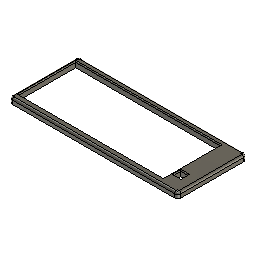
top (Autodesk Fusion 360 design; units mm, degrees)
part number: 2026-03-14-23-38-17-885
Autodesk Fusion 360 part; units mm, degrees
(part 1 of 2)
sketch "Sketch1" plane through (0, 0, 0) normal (0, 0, 1) x (1, 0, 0)
  line L0 (27.4732, 9.3182) -> (40.4732, 9.3182)
  line L1 (-101.1143, 52.4682) -> (-88.1143, 52.4682)
  line L2 (-96.3518, -9.7318) -> (-83.3518, -9.7318)
  arc A0 (-75.7081, -29.2818) -> (-76.2081, -28.7818) centre (-76.2081, -29.2818) ccw
  line L3 (127.4857, 66.4682) -> (140.4857, 66.4682)
  line L4 (146.5357, -4.6818) -> (159.5357, -4.6818)
  line L5 (160.0357, 8.8182) -> (160.0357, -4.1818)
  arc A1 (-40.4893, 14.3682) -> (-39.9893, 14.8682) centre (-40.4893, 14.8682) ccw
  line L6 (75.0982, -23.7318) -> (88.0982, -23.7318)
  arc A2 (146.5357, -28.7818) -> (146.0357, -29.2818) centre (146.5357, -29.2818) ccw
  arc A3 (140.9857, 65.9682) -> (140.4857, 66.4682) centre (140.4857, 65.9682) ccw
  line L7 (146.5357, -9.7318) -> (159.5357, -9.7318)
  arc A4 (36.2107, 27.8682) -> (35.7107, 28.3682) centre (35.7107, 27.8682) ccw
  arc A5 (-45.2518, -23.7318) -> (-44.7518, -23.2318) centre (-45.2518, -23.2318) ccw
  arc A6 (50.4982, -10.2318) -> (49.9982, -9.7318) centre (49.9982, -10.2318) ccw
  arc A7 (17.9482, -9.7318) -> (17.4482, -10.2318) centre (17.9482, -10.2318) ccw
  line L8 (3.6607, 28.3682) -> (16.6607, 28.3682)
  line L9 (8.4232, -4.6818) -> (21.4232, -4.6818)
  line L10 (13.1857, 47.4182) -> (26.1857, 47.4182)
  line L11 (13.1857, 33.4182) -> (26.1857, 33.4182)
  line L12 (3.6607, 14.3682) -> (16.6607, 14.3682)
  line L13 (212.5639, -64.1628) -> (-153.6501, -64.1628)
  line L14 (-153.6501, 86.0492) -> (212.5639, 86.0492)
  line L15 (187.5639, -17.1628) -> (187.5639, -32.1628)
  arc A8 (-44.7518, -10.2318) -> (-45.2518, -9.7318) centre (-45.2518, -10.2318) ccw
  arc A9 (-39.7018, -23.2318) -> (-39.2018, -23.7318) centre (-39.2018, -23.2318) ccw
  line L16 (70.3357, -42.7818) -> (83.3357, -42.7818)
  arc A10 (115.5794, 9.3182) -> (115.0794, 8.8182) centre (115.5794, 8.8182) ccw
  arc A11 (146.5357, 47.4182) -> (146.0357, 46.9182) centre (146.5357, 46.9182) ccw
  line L17 (172.5639, -32.1628) -> (172.5639, -17.1628)
  line L18 (26.6857, 46.9182) -> (26.6857, 33.9182)
  arc A12 (-49.2268, -4.1818) -> (-48.7268, -4.6818) centre (-48.7268, -4.1818) ccw
  circle A13 centre (207.0639, 80.5492) radius 1.45
  line L19 (-30.4643, 46.9182) -> (-30.4643, 33.9182)
  line L20 (3.6607, 52.4682) -> (16.6607, 52.4682)
  line L21 (3.6607, 66.4682) -> (16.6607, 66.4682)
  line L22 (-96.3518, -23.7318) -> (-83.3518, -23.7318)
  line L23 (-111.8701, -25.7318) -> (-105.8701, -25.7318)
  line L24 (-113.8081, -10.2318) -> (-113.8081, -23.2318)
  arc A14 (12.6857, 33.9182) -> (13.1857, 33.4182) centre (13.1857, 33.9182) ccw
  arc A15 (-89.2081, -28.7818) -> (-89.7081, -29.2818) centre (-89.2081, -29.2818) ccw
  arc A16 (-35.7268, -4.6818) -> (-35.2268, -4.1818) centre (-35.7268, -4.1818) ccw
  arc A17 (-15.3893, 28.3682) -> (-15.8893, 27.8682) centre (-15.3893, 27.8682) ccw
  line L25 (-6.3643, 46.9182) -> (-6.3643, 33.9182)
  line L26 (-136.2461, -11.2318) -> (-136.2461, -25.2318)
  line L27 (60.8107, 28.3682) -> (73.8107, 28.3682)
  arc A18 (-88.1143, 33.4182) -> (-87.6143, 33.9182) centre (-88.1143, 33.9182) ccw
  line L28 (69.8357, 46.9182) -> (69.8357, 33.9182)
  arc A19 (-39.2018, -9.7318) -> (-39.7018, -10.2318) centre (-39.2018, -10.2318) ccw
  line L29 (-44.4643, 46.9182) -> (-44.4643, 33.9182)
  arc A20 (-96.8518, -23.2318) -> (-96.3518, -23.7318) centre (-96.3518, -23.2318) ccw
  line L30 (-82.5643, 65.9682) -> (-82.5643, 52.9682)
  line L31 (101.2919, -23.7318) -> (114.2919, -23.7318)
  arc A21 (93.3607, 27.8682) -> (92.8607, 28.3682) centre (92.8607, 27.8682) ccw
  arc A22 (-123.3331, -29.2818) -> (-123.8331, -28.7818) centre (-123.8331, -29.2818) ccw
  line L32 (55.2607, 65.9682) -> (55.2607, 52.9682)
  arc A23 (-30.9643, 33.4182) -> (-30.4643, 33.9182) centre (-30.9643, 33.9182) ccw
  arc A24 (51.2857, 47.4182) -> (50.7857, 46.9182) centre (51.2857, 46.9182) ccw
  line L33 (-30.1768, 8.8182) -> (-30.1768, -4.1818)
  line L34 (88.8857, 65.9682) -> (88.8857, 52.9682)
  line L35 (-129.2461, -11.2318) -> (-129.2461, -25.2318)
  line L36 (-112.3701, -11.2318) -> (-112.3701, -25.2318)
  circle A25 centre (-148.1501, -58.6628) radius 1.45
  arc A26 (17.1607, 27.8682) -> (16.6607, 28.3682) centre (16.6607, 27.8682) ccw
  arc A27 (-106.3768, -4.1818) -> (-105.8768, -4.6818) centre (-105.8768, -4.1818) ccw
  arc A28 (-54.7768, -4.6818) -> (-54.2768, -4.1818) centre (-54.7768, -4.1818) ccw
  arc A29 (-50.0143, 33.4182) -> (-49.5143, 33.9182) centre (-50.0143, 33.9182) ccw
  line L37 (-86.8268, 9.3182) -> (-73.8268, 9.3182)
  arc A30 (127.4857, 66.4682) -> (126.9857, 65.9682) centre (127.4857, 65.9682) ccw
  arc A31 (7.6357, 46.9182) -> (7.1357, 47.4182) centre (7.1357, 46.9182) ccw
  line L38 (-106.6643, 46.9182) -> (-106.6643, 33.9182)
  arc A32 (89.3857, 47.4182) -> (88.8857, 46.9182) centre (89.3857, 46.9182) ccw
  arc A33 (160.0357, -29.2818) -> (159.5357, -28.7818) centre (159.5357, -29.2818) ccw
  arc A34 (106.6414, -6.1818) -> (107.1414, -6.6818) centre (107.1414, -6.1818) ccw
  line L39 (127.4857, 52.4682) -> (140.4857, 52.4682)
  arc A35 (-77.3018, -9.7318) -> (-77.8018, -10.2318) centre (-77.3018, -10.2318) ccw
  line L40 (40.9732, 8.8182) -> (40.9732, -4.1818)
  line L41 (8.4232, 9.3182) -> (21.4232, 9.3182)
  arc A36 (26.9732, -4.1818) -> (27.4732, -4.6818) centre (27.4732, -4.1818) ccw
  arc A37 (40.9732, 8.8182) -> (40.4732, 9.3182) centre (40.4732, 8.8182) ccw
  arc A38 (-111.8701, -10.7318) -> (-112.3701, -11.2318) centre (-111.8701, -11.2318) ccw
  line L42 (-134.9518, 27.8682) -> (-134.9518, 14.8682)
  arc A39 (-35.2268, 8.8182) -> (-35.7268, 9.3182) centre (-35.7268, 8.8182) ccw
  arc A40 (-120.6643, 33.9182) -> (-120.1643, 33.4182) centre (-120.1643, 33.9182) ccw
  arc A41 (-64.3018, -23.7318) -> (-63.8018, -23.2318) centre (-64.3018, -23.2318) ccw
  arc A42 (-43.9643, 47.4182) -> (-44.4643, 46.9182) centre (-43.9643, 46.9182) ccw
  arc A43 (-101.1143, 66.4682) -> (-101.6143, 65.9682) centre (-101.1143, 65.9682) ccw
  arc A44 (-134.9518, 14.8682) -> (-134.4518, 14.3682) centre (-134.4518, 14.8682) ccw
  arc A45 (-113.8081, -10.2318) -> (-114.3081, -9.7318) centre (-114.3081, -10.2318) ccw
  line L43 (17.1607, 65.9682) -> (17.1607, 52.9682)
  arc A46 (7.1357, 33.4182) -> (7.6357, 33.9182) centre (7.1357, 33.9182) ccw
  arc A47 (-53.4893, 28.3682) -> (-53.9893, 27.8682) centre (-53.4893, 27.8682) ccw
  line L44 (-111.8701, -10.7318) -> (-105.8701, -10.7318)
  arc A48 (98.1232, 8.8182) -> (97.6232, 9.3182) centre (97.6232, 8.8182) ccw
  arc A49 (-125.7143, 65.9682) -> (-126.2143, 66.4682) centre (-126.2143, 65.9682) ccw
  arc A50 (108.4357, -28.7818) -> (107.9357, -29.2818) centre (108.4357, -29.2818) ccw
  line L45 (-15.3893, 66.4682) -> (-2.3893, 66.4682)
  line L46 (-101.6143, 65.9682) -> (-101.6143, 52.9682)
  arc A51 (79.8607, 28.3682) -> (79.3607, 27.8682) centre (79.8607, 27.8682) ccw
  line L47 (-44.4643, 65.9682) -> (-44.4643, 52.9682)
  arc A52 (-63.5143, 33.9182) -> (-63.0143, 33.4182) centre (-63.0143, 33.9182) ccw
  line L48 (-78.0893, 27.8682) -> (-78.0893, 14.8682)
  arc A53 (17.1607, 65.9682) -> (16.6607, 66.4682) centre (16.6607, 65.9682) ccw
  line L49 (-53.4893, 28.3682) -> (-40.4893, 28.3682)
  line L50 (-89.2081, -42.7818) -> (-76.2081, -42.7818)
  arc A54 (-64.2706, -29.7818) -> (-64.7706, -30.2818) centre (-64.2706, -30.2818) ccw
  arc A55 (88.8857, 52.9682) -> (89.3857, 52.4682) centre (89.3857, 52.9682) ccw
  arc A56 (-50.0143, 52.4682) -> (-49.5143, 52.9682) centre (-50.0143, 52.9682) ccw
  line L51 (-43.9643, 66.4682) -> (-30.9643, 66.4682)
  line L52 (-82.0643, 52.4682) -> (-69.0643, 52.4682)
  line L53 (-139.2143, 66.4682) -> (-126.2143, 66.4682)
  arc A57 (-15.8893, 52.9682) -> (-15.3893, 52.4682) centre (-15.3893, 52.9682) ccw
  arc A58 (55.2607, 65.9682) -> (54.7607, 66.4682) centre (54.7607, 65.9682) ccw
  line L54 (-73.0393, 27.8682) -> (-73.0393, 14.8682)
  arc A59 (-24.9143, 47.4182) -> (-25.4143, 46.9182) centre (-24.9143, 46.9182) ccw
  arc A60 (83.3357, 33.4182) -> (83.8357, 33.9182) centre (83.3357, 33.9182) ccw
  arc A61 (-120.1643, 47.4182) -> (-120.6643, 46.9182) centre (-120.1643, 46.9182) ccw
  line L55 (-139.2143, 47.4182) -> (-126.2143, 47.4182)
  arc A62 (-72.5393, 28.3682) -> (-73.0393, 27.8682) centre (-72.5393, 27.8682) ccw
  line L56 (-63.5143, 65.9682) -> (-63.5143, 52.9682)
  arc A63 (-82.5643, 33.9182) -> (-82.0643, 33.4182) centre (-82.0643, 33.9182) ccw
  line L57 (-139.7143, 65.9682) -> (-139.7143, 52.9682)
  arc A64 (-97.6393, 14.3682) -> (-97.1393, 14.8682) centre (-97.6393, 14.8682) ccw
  circle A65 centre (-148.1501, 80.5492) radius 1.45
  arc A66 (-68.5643, 46.9182) -> (-69.0643, 47.4182) centre (-69.0643, 46.9182) ccw
  line L58 (-82.0643, 47.4182) -> (-69.0643, 47.4182)
  arc A67 (-111.1393, 14.8682) -> (-110.6393, 14.3682) centre (-110.6393, 14.8682) ccw
  line L59 (7.6357, 46.9182) -> (7.6357, 33.9182)
  arc A68 (-49.5143, 65.9682) -> (-50.0143, 66.4682) centre (-50.0143, 65.9682) ccw
  arc A69 (-106.6643, 46.9182) -> (-107.1643, 47.4182) centre (-107.1643, 46.9182) ccw
  arc A70 (-20.9393, 27.8682) -> (-21.4393, 28.3682) centre (-21.4393, 27.8682) ccw
  arc A71 (-6.3643, 33.9182) -> (-5.8643, 33.4182) centre (-5.8643, 33.9182) ccw
  arc A72 (69.8357, 33.9182) -> (70.3357, 33.4182) centre (70.3357, 33.9182) ccw
  arc A73 (-107.1643, 33.4182) -> (-106.6643, 33.9182) centre (-107.1643, 33.9182) ccw
  arc A74 (7.9232, -4.1818) -> (8.4232, -4.6818) centre (8.4232, -4.1818) ccw
  arc A75 (55.5482, -23.2318) -> (56.0482, -23.7318) centre (56.0482, -23.2318) ccw
  arc A76 (51.2857, -28.7818) -> (50.7857, -29.2818) centre (51.2857, -29.2818) ccw
  arc A77 (-16.1768, 8.8182) -> (-16.6768, 9.3182) centre (-16.6768, 8.8182) ccw
  line L60 (35.7294, -44.7818) -> (41.7294, -44.7818)
  arc A78 (-21.4393, 14.3682) -> (-20.9393, 14.8682) centre (-21.4393, 14.8682) ccw
  line L61 (17.9482, -23.7318) -> (30.9482, -23.7318)
  line L62 (-16.1768, 8.8182) -> (-16.1768, -4.1818)
  line L63 (42.2294, -30.2818) -> (42.2294, -44.2818)
  arc A79 (-10.6268, 9.3182) -> (-11.1268, 8.8182) centre (-10.6268, 8.8182) ccw
  line L64 (84.6232, -4.6818) -> (97.6232, -4.6818)
  arc A80 (49.9982, -23.7318) -> (50.4982, -23.2318) centre (49.9982, -23.2318) ccw
  arc A81 (36.4982, -23.2318) -> (36.9982, -23.7318) centre (36.9982, -23.2318) ccw
  arc A82 (-6.6518, -10.2318) -> (-7.1518, -9.7318) centre (-7.1518, -10.2318) ccw
  line L65 (89.3857, 33.4182) -> (102.3857, 33.4182)
  line L66 (-67.7768, -4.6818) -> (-54.7768, -4.6818)
  line L67 (26.9732, 8.8182) -> (26.9732, -4.1818)
  arc A83 (31.4482, -10.2318) -> (30.9482, -9.7318) centre (30.9482, -10.2318) ccw
  arc A84 (46.5232, 9.3182) -> (46.0232, 8.8182) centre (46.5232, 8.8182) ccw
  arc A85 (22.2107, 14.8682) -> (22.7107, 14.3682) centre (22.7107, 14.8682) ccw
  line L68 (21.9232, 8.8182) -> (21.9232, -4.1818)
  line L69 (-135.7461, -25.7318) -> (-129.7461, -25.7318)
  arc A86 (64.2857, 33.4182) -> (64.7857, 33.9182) centre (64.2857, 33.9182) ccw
  arc A87 (-83.3518, -23.7318) -> (-82.8518, -23.2318) centre (-83.3518, -23.2318) ccw
  line L70 (-123.3331, -29.2818) -> (-123.3331, -42.2818)
  line L71 (-136.8331, -28.7818) -> (-123.8331, -28.7818)
  arc A88 (-89.7081, -42.2818) -> (-89.2081, -42.7818) centre (-89.2081, -42.2818) ccw
  line L72 (-127.8081, -10.2318) -> (-127.8081, -23.2318)
  arc A89 (89.3857, 66.4682) -> (88.8857, 65.9682) centre (89.3857, 65.9682) ccw
  arc A90 (101.2919, -9.7318) -> (100.7919, -10.2318) centre (101.2919, -10.2318) ccw
  arc A91 (41.7607, 66.4682) -> (41.2607, 65.9682) centre (41.7607, 65.9682) ccw
  line L73 (-82.0643, 66.4682) -> (-69.0643, 66.4682)
  arc A92 (-30.4643, 65.9682) -> (-30.9643, 66.4682) centre (-30.9643, 65.9682) ccw
  line L74 (-139.2143, 52.4682) -> (-126.2143, 52.4682)
  line L75 (-120.1643, 47.4182) -> (-107.1643, 47.4182)
  line L76 (22.2107, 65.9682) -> (22.2107, 52.9682)
  arc A93 (-29.6768, 9.3182) -> (-30.1768, 8.8182) centre (-29.6768, 8.8182) ccw
  line L77 (-110.6393, 28.3682) -> (-97.6393, 28.3682)
  arc A94 (-105.8768, 9.3182) -> (-106.3768, 8.8182) centre (-105.8768, 8.8182) ccw
  arc A95 (54.7607, 52.4682) -> (55.2607, 52.9682) centre (54.7607, 52.9682) ccw
  line L78 (-48.7268, 9.3182) -> (-35.7268, 9.3182)
  line L79 (-92.0893, 27.8682) -> (-92.0893, 14.8682)
  line L80 (-1.8893, 65.9682) -> (-1.8893, 52.9682)
  arc A96 (-76.2081, -42.7818) -> (-75.7081, -42.2818) centre (-76.2081, -42.2818) ccw
  arc A97 (-49.5143, 46.9182) -> (-50.0143, 47.4182) centre (-50.0143, 46.9182) ccw
  arc A98 (-129.2461, -11.2318) -> (-129.7461, -10.7318) centre (-129.7461, -11.2318) ccw
  arc A99 (-44.4643, 33.9182) -> (-43.9643, 33.4182) centre (-43.9643, 33.9182) ccw
  line L81 (83.8357, 65.9682) -> (83.8357, 52.9682)
  arc A100 (89.3857, -28.7818) -> (88.8857, -29.2818) centre (89.3857, -29.2818) ccw
  line L82 (-77.3018, -9.7318) -> (-64.3018, -9.7318)
  arc A101 (-135.7461, -10.7318) -> (-136.2461, -11.2318) centre (-135.7461, -11.2318) ccw
  circle A102 centre (207.0639, -58.6628) radius 1.45
  line L83 (22.7107, 28.3682) -> (35.7107, 28.3682)
  line L84 (-11.4143, 46.9182) -> (-11.4143, 33.9182)
  arc A103 (-1.8893, 65.9682) -> (-2.3893, 66.4682) centre (-2.3893, 65.9682) ccw
  arc A104 (70.3357, 47.4182) -> (69.8357, 46.9182) centre (70.3357, 46.9182) ccw
  arc A105 (64.2857, -42.7818) -> (64.7857, -42.2818) centre (64.2857, -42.2818) ccw
  line L85 (-105.3701, -11.2318) -> (-105.3701, -25.2318)
  line L86 (131.0174, -6.6818) -> (137.0174, -6.6818)
  line L87 (-58.2518, -9.7318) -> (-45.2518, -9.7318)
  line L88 (-101.1143, 33.4182) -> (-88.1143, 33.4182)
  line L89 (-120.9518, 27.8682) -> (-120.9518, 14.8682)
  arc A106 (-101.1143, 47.4182) -> (-101.6143, 46.9182) centre (-101.1143, 46.9182) ccw
  line L90 (-139.2143, 33.4182) -> (-126.2143, 33.4182)
  arc A107 (-110.6393, 28.3682) -> (-111.1393, 27.8682) centre (-110.6393, 27.8682) ccw
  line L91 (12.6857, 46.9182) -> (12.6857, 33.9182)
  arc A108 (-82.0643, 66.4682) -> (-82.5643, 65.9682) centre (-82.0643, 65.9682) ccw
  line L92 (-132.0706, 9.3182) -> (-119.0706, 9.3182)
  arc A109 (-120.9518, 27.8682) -> (-121.4518, 28.3682) centre (-121.4518, 27.8682) ccw
  arc A110 (-125.7143, 46.9182) -> (-126.2143, 47.4182) centre (-126.2143, 46.9182) ccw
  arc A111 (-139.7143, 33.9182) -> (-139.2143, 33.4182) centre (-139.2143, 33.9182) ccw
  arc A112 (-97.1393, 27.8682) -> (-97.6393, 28.3682) centre (-97.6393, 27.8682) ccw
  arc A113 (-2.3893, 14.3682) -> (-1.8893, 14.8682) centre (-2.3893, 14.8682) ccw
  arc A114 (35.2294, -44.2818) -> (35.7294, -44.7818) centre (35.7294, -44.2818) ccw
  arc A115 (-11.1268, -4.1818) -> (-10.6268, -4.6818) centre (-10.6268, -4.1818) ccw
  arc A116 (50.7857, -42.2818) -> (51.2857, -42.7818) centre (51.2857, -42.2818) ccw
  line L93 (41.7607, 14.3682) -> (54.7607, 14.3682)
  arc A117 (35.7294, -29.7818) -> (35.2294, -30.2818) centre (35.7294, -30.2818) ccw
  arc A118 (-20.1518, -9.7318) -> (-20.6518, -10.2318) centre (-20.1518, -10.2318) ccw
  arc A119 (8.4232, 9.3182) -> (7.9232, 8.8182) centre (8.4232, 8.8182) ccw
  line L94 (35.2294, -30.2818) -> (35.2294, -44.2818)
  line L95 (89.3857, 66.4682) -> (102.3857, 66.4682)
  line L96 (-1.1018, -9.7318) -> (11.8982, -9.7318)
  line L97 (36.9982, -23.7318) -> (49.9982, -23.7318)
  line L98 (36.4982, -10.2318) -> (36.4982, -23.2318)
  line L99 (55.5482, -10.2318) -> (55.5482, -23.2318)
  line L100 (-11.1268, 8.8182) -> (-11.1268, -4.1818)
  line L101 (7.9232, 8.8182) -> (7.9232, -4.1818)
  arc A120 (17.4482, -23.2318) -> (17.9482, -23.7318) centre (17.9482, -23.2318) ccw
  arc A121 (3.1607, 14.8682) -> (3.6607, 14.3682) centre (3.6607, 14.8682) ccw
  line L102 (-15.3893, 14.3682) -> (-2.3893, 14.3682)
  arc A122 (-15.8893, 14.8682) -> (-15.3893, 14.3682) centre (-15.3893, 14.8682) ccw
  line L103 (50.7857, -29.2818) -> (50.7857, -42.2818)
  arc A123 (30.9482, -23.7318) -> (31.4482, -23.2318) centre (30.9482, -23.2318) ccw
  line L104 (27.4732, -4.6818) -> (40.4732, -4.6818)
  line L105 (88.8857, -29.2818) -> (88.8857, -42.2818)
  arc A124 (69.8357, -42.2818) -> (70.3357, -42.7818) centre (70.3357, -42.2818) ccw
  line L106 (-125.7143, 46.9182) -> (-125.7143, 33.9182)
  line L107 (-48.7268, -4.6818) -> (-35.7268, -4.6818)
  arc A125 (3.6607, 66.4682) -> (3.1607, 65.9682) centre (3.6607, 65.9682) ccw
  arc A126 (-68.2768, -4.1818) -> (-67.7768, -4.6818) centre (-67.7768, -4.1818) ccw
  line L108 (146.5357, -42.7818) -> (159.5357, -42.7818)
  arc A127 (-105.3701, -11.2318) -> (-105.8701, -10.7318) centre (-105.8701, -11.2318) ccw
  arc A128 (13.1857, 47.4182) -> (12.6857, 46.9182) centre (13.1857, 46.9182) ccw
  arc A129 (32.2357, 47.4182) -> (31.7357, 46.9182) centre (32.2357, 46.9182) ccw
  arc A130 (113.1414, -6.6818) -> (113.6414, -6.1818) centre (113.1414, -6.1818) ccw
  arc A131 (26.6857, 46.9182) -> (26.1857, 47.4182) centre (26.1857, 46.9182) ccw
  arc A132 (-34.4393, 28.3682) -> (-34.9393, 27.8682) centre (-34.4393, 27.8682) ccw
  line L109 (-68.5643, 46.9182) -> (-68.5643, 33.9182)
  line L110 (127.4857, -23.7318) -> (140.4857, -23.7318)
  arc A133 (83.8357, 46.9182) -> (83.3357, 47.4182) centre (83.3357, 46.9182) ccw
  arc A134 (64.7857, 46.9182) -> (64.2857, 47.4182) centre (64.2857, 46.9182) ccw
  line L111 (108.4357, -42.7818) -> (121.4357, -42.7818)
  arc A135 (140.4857, -42.7818) -> (140.9857, -42.2818) centre (140.4857, -42.2818) ccw
  line L112 (64.7857, -29.2818) -> (64.7857, -42.2818)
  line L113 (146.5357, -28.7818) -> (159.5357, -28.7818)
  arc A136 (-77.8018, -23.2318) -> (-77.3018, -23.7318) centre (-77.3018, -23.2318) ccw
  arc A137 (-99.5206, -29.2818) -> (-100.0206, -28.7818) centre (-100.0206, -29.2818) ccw
  line L114 (-91.5893, 14.3682) -> (-78.5893, 14.3682)
  arc A138 (31.7357, 33.9182) -> (32.2357, 33.4182) centre (32.2357, 33.9182) ccw
  line L115 (-127.3081, -23.7318) -> (-114.3081, -23.7318)
  line L116 (-15.3893, 28.3682) -> (-2.3893, 28.3682)
  arc A139 (-25.4143, 33.9182) -> (-24.9143, 33.4182) centre (-24.9143, 33.9182) ccw
  line L117 (-111.1393, 27.8682) -> (-111.1393, 14.8682)
  arc A140 (-118.5706, 8.8182) -> (-119.0706, 9.3182) centre (-119.0706, 8.8182) ccw
  arc A141 (55.2607, 27.8682) -> (54.7607, 28.3682) centre (54.7607, 27.8682) ccw
  arc A142 (-87.6143, 65.9682) -> (-88.1143, 66.4682) centre (-88.1143, 65.9682) ccw
  line L118 (-120.1643, 33.4182) -> (-107.1643, 33.4182)
  arc A143 (-139.2143, 66.4682) -> (-139.7143, 65.9682) centre (-139.2143, 65.9682) ccw
  arc A144 (-139.7143, 52.9682) -> (-139.2143, 52.4682) centre (-139.2143, 52.9682) ccw
  line L119 (41.2607, 65.9682) -> (41.2607, 52.9682)
  line L120 (69.8357, 65.9682) -> (69.8357, 52.9682)
  arc A145 (-101.6143, 52.9682) -> (-101.1143, 52.4682) centre (-101.1143, 52.9682) ccw
  line L121 (70.3357, 47.4182) -> (83.3357, 47.4182)
  arc A146 (36.2107, 65.9682) -> (35.7107, 66.4682) centre (35.7107, 65.9682) ccw
  arc A147 (3.1607, 52.9682) -> (3.6607, 52.4682) centre (3.6607, 52.9682) ccw
  arc A148 (-82.5643, 52.9682) -> (-82.0643, 52.4682) centre (-82.0643, 52.9682) ccw
  line L122 (22.7107, 52.4682) -> (35.7107, 52.4682)
  line L123 (70.3357, 33.4182) -> (83.3357, 33.4182)
  arc A149 (-15.3893, 66.4682) -> (-15.8893, 65.9682) centre (-15.3893, 65.9682) ccw
  arc A150 (-91.5893, 28.3682) -> (-92.0893, 27.8682) centre (-91.5893, 27.8682) ccw
  arc A151 (-126.2143, 52.4682) -> (-125.7143, 52.9682) centre (-126.2143, 52.9682) ccw
  arc A152 (-132.0706, 9.3182) -> (-132.5706, 8.8182) centre (-132.0706, 8.8182) ccw
  arc A153 (3.6607, 28.3682) -> (3.1607, 27.8682) centre (3.6607, 27.8682) ccw
  arc A154 (-78.0893, 27.8682) -> (-78.5893, 28.3682) centre (-78.5893, 27.8682) ccw
  arc A155 (-30.4643, 46.9182) -> (-30.9643, 47.4182) centre (-30.9643, 46.9182) ccw
  arc A156 (69.8357, 52.9682) -> (70.3357, 52.4682) centre (70.3357, 52.9682) ccw
  arc A157 (-87.6143, 46.9182) -> (-88.1143, 47.4182) centre (-88.1143, 46.9182) ccw
  arc A158 (16.6607, 14.3682) -> (17.1607, 14.8682) centre (16.6607, 14.8682) ccw
  arc A159 (40.4732, -4.6818) -> (40.9732, -4.1818) centre (40.4732, -4.1818) ccw
  arc A160 (27.4732, 9.3182) -> (26.9732, 8.8182) centre (27.4732, 8.8182) ccw
  line L124 (22.7107, 14.3682) -> (35.7107, 14.3682)
  arc A161 (126.9857, -23.2318) -> (127.4857, -23.7318) centre (127.4857, -23.2318) ccw
  arc A162 (-57.7706, -30.2818) -> (-58.2706, -29.7818) centre (-58.2706, -30.2818) ccw
  line L125 (31.7357, 46.9182) -> (31.7357, 33.9182)
  arc A163 (127.4857, -9.7318) -> (126.9857, -10.2318) centre (127.4857, -10.2318) ccw
  line L126 (-58.2518, -23.7318) -> (-45.2518, -23.7318)
  arc A164 (-58.2706, -44.7818) -> (-57.7706, -44.2818) centre (-58.2706, -44.2818) ccw
  line L127 (146.5357, 47.4182) -> (159.5357, 47.4182)
  arc A165 (126.9857, 52.9682) -> (127.4857, 52.4682) centre (127.4857, 52.9682) ccw
  arc A166 (-73.0393, 14.8682) -> (-72.5393, 14.3682) centre (-72.5393, 14.8682) ccw
  arc A167 (70.3357, -28.7818) -> (69.8357, -29.2818) centre (70.3357, -29.2818) ccw
  line L128 (-86.8268, -4.6818) -> (-73.8268, -4.6818)
  line L129 (-54.2768, 8.8182) -> (-54.2768, -4.1818)
  arc A168 (-63.8018, -10.2318) -> (-64.3018, -9.7318) centre (-64.3018, -10.2318) ccw
  arc A169 (-101.6143, 33.9182) -> (-101.1143, 33.4182) centre (-101.1143, 33.9182) ccw
  arc A170 (-63.5143, 52.9682) -> (-63.0143, 52.4682) centre (-63.0143, 52.9682) ccw
  arc A171 (16.6607, 52.4682) -> (17.1607, 52.9682) centre (16.6607, 52.9682) ccw
  line L130 (-97.1393, 27.8682) -> (-97.1393, 14.8682)
  line L131 (-49.5143, 46.9182) -> (-49.5143, 33.9182)
  line L132 (-82.0643, 33.4182) -> (-69.0643, 33.4182)
  arc A172 (-82.0643, 47.4182) -> (-82.5643, 46.9182) centre (-82.0643, 46.9182) ccw
  arc A173 (-126.2143, 33.4182) -> (-125.7143, 33.9182) centre (-126.2143, 33.9182) ccw
  arc A174 (-64.7706, -44.2818) -> (-64.2706, -44.7818) centre (-64.2706, -44.2818) ccw
  arc A175 (-11.9143, 33.4182) -> (-11.4143, 33.9182) centre (-11.9143, 33.9182) ccw
  line L133 (-134.4518, 28.3682) -> (-121.4518, 28.3682)
  line L134 (-43.9643, 52.4682) -> (-30.9643, 52.4682)
  arc A176 (-92.3768, 8.8182) -> (-92.8768, 9.3182) centre (-92.8768, 8.8182) ccw
  line L135 (22.7107, 66.4682) -> (35.7107, 66.4682)
  line L136 (-5.8643, 33.4182) -> (7.1357, 33.4182)
  line L137 (70.3357, 66.4682) -> (83.3357, 66.4682)
  line L138 (-43.9643, 47.4182) -> (-30.9643, 47.4182)
  line L139 (-89.7081, -29.2818) -> (-89.7081, -42.2818)
  line L140 (64.7857, 46.9182) -> (64.7857, 33.9182)
  arc A177 (-139.2143, 47.4182) -> (-139.7143, 46.9182) centre (-139.2143, 46.9182) ccw
  arc A178 (-63.0143, 47.4182) -> (-63.5143, 46.9182) centre (-63.0143, 46.9182) ccw
  line L141 (3.1607, 65.9682) -> (3.1607, 52.9682)
  arc A179 (-78.5893, 14.3682) -> (-78.0893, 14.8682) centre (-78.5893, 14.8682) ccw
  line L142 (107.9357, -29.2818) -> (107.9357, -42.2818)
  line L143 (-135.7461, -10.7318) -> (-129.7461, -10.7318)
  arc A180 (60.8107, 28.3682) -> (60.3107, 27.8682) centre (60.8107, 27.8682) ccw
  arc A181 (35.7107, 52.4682) -> (36.2107, 52.9682) centre (35.7107, 52.9682) ccw
  line L144 (46.0232, 8.8182) -> (46.0232, -4.1818)
  arc A182 (35.7107, 14.3682) -> (36.2107, 14.8682) centre (35.7107, 14.8682) ccw
  line L145 (101.2919, -9.7318) -> (114.2919, -9.7318)
  arc A183 (102.3857, -42.7818) -> (102.8857, -42.2818) centre (102.3857, -42.2818) ccw
  line L146 (146.5357, -23.7318) -> (159.5357, -23.7318)
  arc A184 (-82.8518, -10.2318) -> (-83.3518, -9.7318) centre (-83.3518, -10.2318) ccw
  arc A185 (-119.0706, -4.6818) -> (-118.5706, -4.1818) centre (-119.0706, -4.1818) ccw
  arc A186 (-136.8331, -28.7818) -> (-137.3331, -29.2818) centre (-136.8331, -29.2818) ccw
  arc A187 (140.4857, 52.4682) -> (140.9857, 52.9682) centre (140.4857, 52.9682) ccw
  line L147 (70.3357, -28.7818) -> (83.3357, -28.7818)
  line L148 (-113.5206, -29.2818) -> (-113.5206, -42.2818)
  arc A188 (22.7107, 28.3682) -> (22.2107, 27.8682) centre (22.7107, 27.8682) ccw
  arc A189 (-54.2768, 8.8182) -> (-54.7768, 9.3182) centre (-54.7768, 8.8182) ccw
  arc A190 (64.7857, -29.2818) -> (64.2857, -28.7818) centre (64.2857, -29.2818) ccw
  line L149 (115.0794, 8.8182) -> (115.0794, -4.1818)
  arc A191 (-123.8331, -42.7818) -> (-123.3331, -42.2818) centre (-123.8331, -42.2818) ccw
  arc A192 (-1.8893, 27.8682) -> (-2.3893, 28.3682) centre (-2.3893, 27.8682) ccw
  arc A193 (-132.5706, -4.1818) -> (-132.0706, -4.6818) centre (-132.0706, -4.1818) ccw
  arc A194 (-2.3893, 52.4682) -> (-1.8893, 52.9682) centre (-2.3893, 52.9682) ccw
  arc A195 (-59.0393, 27.8682) -> (-59.5393, 28.3682) centre (-59.5393, 27.8682) ccw
  arc A196 (-113.0206, -28.7818) -> (-113.5206, -29.2818) centre (-113.0206, -29.2818) ccw
  arc A197 (45.7357, 46.9182) -> (45.2357, 47.4182) centre (45.2357, 46.9182) ccw
  arc A198 (-100.0206, -42.7818) -> (-99.5206, -42.2818) centre (-100.0206, -42.2818) ccw
  arc A199 (-127.3081, -9.7318) -> (-127.8081, -10.2318) centre (-127.3081, -10.2318) ccw
  line L150 (-49.2268, 8.8182) -> (-49.2268, -4.1818)
  arc A200 (140.4857, -23.7318) -> (140.9857, -23.2318) centre (140.4857, -23.2318) ccw
  arc A201 (-59.5393, 14.3682) -> (-59.0393, 14.8682) centre (-59.5393, 14.8682) ccw
  arc A202 (26.1857, 33.4182) -> (26.6857, 33.9182) centre (26.1857, 33.9182) ccw
  arc A203 (-11.4143, 46.9182) -> (-11.9143, 47.4182) centre (-11.9143, 46.9182) ccw
  line L151 (-63.5143, 46.9182) -> (-63.5143, 33.9182)
  arc A204 (-127.8081, -23.2318) -> (-127.3081, -23.7318) centre (-127.3081, -23.2318) ccw
  line L152 (102.8857, -29.2818) -> (102.8857, -42.2818)
  arc A205 (114.7919, -10.2318) -> (114.2919, -9.7318) centre (114.2919, -10.2318) ccw
  arc A206 (-58.2518, -9.7318) -> (-58.7518, -10.2318) centre (-58.2518, -10.2318) ccw
  arc A207 (-113.5206, -42.2818) -> (-113.0206, -42.7818) centre (-113.0206, -42.2818) ccw
  line L153 (-99.5206, -29.2818) -> (-99.5206, -42.2818)
  arc A208 (-67.7768, 9.3182) -> (-68.2768, 8.8182) centre (-67.7768, 8.8182) ccw
  line L154 (-87.6143, 46.9182) -> (-87.6143, 33.9182)
  line L155 (-82.5643, 46.9182) -> (-82.5643, 33.9182)
  line L156 (-120.6643, 46.9182) -> (-120.6643, 33.9182)
  arc A209 (159.5357, -23.7318) -> (160.0357, -23.2318) centre (159.5357, -23.2318) ccw
  line L157 (-137.3331, -29.2818) -> (-137.3331, -42.2818)
  arc A210 (74.3107, 27.8682) -> (73.8107, 28.3682) centre (73.8107, 27.8682) ccw
  line L158 (-49.5143, 65.9682) -> (-49.5143, 52.9682)
  line L159 (36.2107, 65.9682) -> (36.2107, 52.9682)
  line L160 (79.8607, 28.3682) -> (92.8607, 28.3682)
  arc A211 (22.7107, 66.4682) -> (22.2107, 65.9682) centre (22.7107, 65.9682) ccw
  line L161 (-125.7143, 65.9682) -> (-125.7143, 52.9682)
  arc A212 (-134.4518, 28.3682) -> (-134.9518, 27.8682) centre (-134.4518, 27.8682) ccw
  arc A213 (-5.8643, 47.4182) -> (-6.3643, 46.9182) centre (-5.8643, 46.9182) ccw
  arc A214 (-121.4518, 14.3682) -> (-120.9518, 14.8682) centre (-121.4518, 14.8682) ccw
  arc A215 (-88.1143, 52.4682) -> (-87.6143, 52.9682) centre (-88.1143, 52.9682) ccw
  line L162 (-68.5643, 65.9682) -> (-68.5643, 52.9682)
  line L163 (-110.6393, 14.3682) -> (-97.6393, 14.3682)
  line L164 (70.3357, 52.4682) -> (83.3357, 52.4682)
  line L165 (-134.4518, 14.3682) -> (-121.4518, 14.3682)
  arc A216 (88.8857, 33.9182) -> (89.3857, 33.4182) centre (89.3857, 33.9182) ccw
  arc A217 (41.2607, 52.9682) -> (41.7607, 52.4682) centre (41.7607, 52.9682) ccw
  line L166 (88.8857, 46.9182) -> (88.8857, 33.9182)
  line L167 (83.8357, 46.9182) -> (83.8357, 33.9182)
  line L168 (-5.8643, 47.4182) -> (7.1357, 47.4182)
  arc A218 (-43.9643, 66.4682) -> (-44.4643, 65.9682) centre (-43.9643, 65.9682) ccw
  arc A219 (22.2107, 52.9682) -> (22.7107, 52.4682) centre (22.7107, 52.9682) ccw
  line L169 (113.6414, 7.8182) -> (113.6414, -6.1818)
  arc A220 (-63.0143, 66.4682) -> (-63.5143, 65.9682) centre (-63.0143, 65.9682) ccw
  arc A221 (-69.0643, 52.4682) -> (-68.5643, 52.9682) centre (-69.0643, 52.9682) ccw
  line L170 (-87.6143, 65.9682) -> (-87.6143, 52.9682)
  line L171 (-91.5893, 28.3682) -> (-78.5893, 28.3682)
  arc A222 (70.3357, 66.4682) -> (69.8357, 65.9682) centre (70.3357, 65.9682) ccw
  line L172 (-64.7706, -30.2818) -> (-64.7706, -44.2818)
  line L173 (32.2357, 47.4182) -> (45.2357, 47.4182)
  arc A223 (83.8357, 65.9682) -> (83.3357, 66.4682) centre (83.3357, 65.9682) ccw
  arc A224 (-53.9893, 14.8682) -> (-53.4893, 14.3682) centre (-53.4893, 14.8682) ccw
  line L174 (-136.8331, -42.7818) -> (-123.8331, -42.7818)
  line L175 (-127.3081, -9.7318) -> (-114.3081, -9.7318)
  arc A225 (121.4357, -42.7818) -> (121.9357, -42.2818) centre (121.4357, -42.2818) ccw
  arc A226 (83.3357, 52.4682) -> (83.8357, 52.9682) centre (83.3357, 52.9682) ccw
  line L176 (-25.4143, 46.9182) -> (-25.4143, 33.9182)
  arc A227 (-25.7018, -10.2318) -> (-26.2018, -9.7318) centre (-26.2018, -10.2318) ccw
  arc A228 (-86.8268, 9.3182) -> (-87.3268, 8.8182) centre (-86.8268, 8.8182) ccw
  arc A229 (-92.0893, 14.8682) -> (-91.5893, 14.3682) centre (-91.5893, 14.8682) ccw
  arc A230 (-73.3268, 8.8182) -> (-73.8268, 9.3182) centre (-73.8268, 8.8182) ccw
  arc A231 (-68.5643, 65.9682) -> (-69.0643, 66.4682) centre (-69.0643, 65.9682) ccw
  line L177 (-101.6143, 46.9182) -> (-101.6143, 33.9182)
  line L178 (-89.2081, -28.7818) -> (-76.2081, -28.7818)
  arc A232 (-137.3331, -42.2818) -> (-136.8331, -42.7818) centre (-136.8331, -42.2818) ccw
  line L179 (-75.7081, -29.2818) -> (-75.7081, -42.2818)
  line L180 (-30.4643, 65.9682) -> (-30.4643, 52.9682)
  line L181 (-15.3893, 52.4682) -> (-2.3893, 52.4682)
  arc A233 (-69.0643, 33.4182) -> (-68.5643, 33.9182) centre (-69.0643, 33.9182) ccw
  arc A234 (-114.3081, -23.7318) -> (-113.8081, -23.2318) centre (-114.3081, -23.2318) ccw
  arc A235 (-48.7268, 9.3182) -> (-49.2268, 8.8182) centre (-48.7268, 8.8182) ccw
  line L182 (-132.0706, -4.6818) -> (-119.0706, -4.6818)
  line L183 (-139.7143, 46.9182) -> (-139.7143, 33.9182)
  line L184 (-77.3018, -23.7318) -> (-64.3018, -23.7318)
  line L185 (106.6414, 7.8182) -> (106.6414, -6.1818)
  line L186 (17.9482, -9.7318) -> (30.9482, -9.7318)
  arc A236 (21.9232, 8.8182) -> (21.4232, 9.3182) centre (21.4232, 8.8182) ccw
  arc A237 (54.7607, 14.3682) -> (55.2607, 14.8682) centre (54.7607, 14.8682) ccw
  arc A238 (36.9982, -9.7318) -> (36.4982, -10.2318) centre (36.9982, -10.2318) ccw
  arc A239 (41.2607, 14.8682) -> (41.7607, 14.3682) centre (41.7607, 14.8682) ccw
  arc A240 (-16.6768, -4.6818) -> (-16.1768, -4.1818) centre (-16.6768, -4.1818) ccw
  arc A241 (42.2294, -30.2818) -> (41.7294, -29.7818) centre (41.7294, -30.2818) ccw
  arc A242 (2.8732, 8.8182) -> (2.3732, 9.3182) centre (2.3732, 8.8182) ccw
  arc A243 (41.7294, -44.7818) -> (42.2294, -44.2818) centre (41.7294, -44.2818) ccw
  line L187 (35.7294, -29.7818) -> (41.7294, -29.7818)
  arc A244 (-1.1018, -9.7318) -> (-1.6018, -10.2318) centre (-1.1018, -10.2318) ccw
  line L188 (69.5482, -10.2318) -> (69.5482, -23.2318)
  arc A245 (112.4107, 27.8682) -> (111.9107, 28.3682) centre (111.9107, 27.8682) ccw
  line L189 (74.5982, -10.2318) -> (74.5982, -23.2318)
  line L190 (-44.7518, -10.2318) -> (-44.7518, -23.2318)
  line L191 (127.4857, -9.7318) -> (140.4857, -9.7318)
  line L192 (-58.7518, -10.2318) -> (-58.7518, -23.2318)
  line L193 (146.5357, 28.3682) -> (159.5357, 28.3682)
  arc A246 (146.5357, 28.3682) -> (146.0357, 27.8682) centre (146.5357, 27.8682) ccw
  arc A247 (107.9357, -42.2818) -> (108.4357, -42.7818) centre (108.4357, -42.2818) ccw
  line L194 (160.0357, 27.8682) -> (160.0357, 14.8682)
  arc A248 (146.5357, -9.7318) -> (146.0357, -10.2318) centre (146.5357, -10.2318) ccw
  arc A249 (102.8857, 46.9182) -> (102.3857, 47.4182) centre (102.3857, 46.9182) ccw
  line L195 (-113.0206, -42.7818) -> (-100.0206, -42.7818)
  line L196 (107.1414, -6.6818) -> (113.1414, -6.6818)
  arc A250 (146.0357, 33.9182) -> (146.5357, 33.4182) centre (146.5357, 33.9182) ccw
  arc A251 (159.5357, 14.3682) -> (160.0357, 14.8682) centre (159.5357, 14.8682) ccw
  arc A252 (131.0174, 8.3182) -> (130.5174, 7.8182) centre (131.0174, 7.8182) ccw
  arc A253 (122.7232, 28.3682) -> (122.2232, 27.8682) centre (122.7232, 27.8682) ccw
  line L197 (-25.7018, -10.2318) -> (-25.7018, -23.2318)
  arc A254 (116.0227, 45.9182) -> (115.5227, 46.4182) centre (115.5227, 45.9182) ccw
  line L198 (-153.6501, -64.1628) -> (-153.6501, 86.0492)
  line L199 (102.8857, 65.9682) -> (102.8857, 52.9682)
  line L200 (140.9857, -29.2818) -> (140.9857, -42.2818)
  line L201 (98.9107, 14.3682) -> (111.9107, 14.3682)
  line L202 (98.4107, 27.8682) -> (98.4107, 14.8682)
  arc A255 (160.0357, 46.9182) -> (159.5357, 47.4182) centre (159.5357, 46.9182) ccw
  arc A256 (130.9607, 33.4182) -> (131.4607, 33.9182) centre (130.9607, 33.9182) ccw
  arc A257 (75.0982, -9.7318) -> (74.5982, -10.2318) centre (75.0982, -10.2318) ccw
  arc A258 (146.0357, -4.1818) -> (146.5357, -4.6818) centre (146.5357, -4.1818) ccw
  arc A259 (146.5357, 9.3182) -> (146.0357, 8.8182) centre (146.5357, 8.8182) ccw
  line L203 (-39.7018, -10.2318) -> (-39.7018, -23.2318)
  arc A260 (122.2232, 14.8682) -> (122.7232, 14.3682) centre (122.7232, 14.8682) ccw
  arc A261 (-44.4643, 52.9682) -> (-43.9643, 52.4682) centre (-43.9643, 52.9682) ccw
  arc A262 (109.0227, 31.9182) -> (109.5227, 31.4182) centre (109.5227, 31.9182) ccw
  arc A263 (140.9857, -29.2818) -> (140.4857, -28.7818) centre (140.4857, -29.2818) ccw
  line L204 (51.2857, 47.4182) -> (64.2857, 47.4182)
  line L205 (-101.1143, 66.4682) -> (-88.1143, 66.4682)
  arc A264 (102.3857, 33.4182) -> (102.8857, 33.9182) centre (102.3857, 33.9182) ccw
  arc A265 (133.3987, 46.4182) -> (132.8987, 45.9182) centre (133.3987, 45.9182) ccw
  line L206 (-43.9643, 33.4182) -> (-30.9643, 33.4182)
  arc A266 (139.3987, 31.4182) -> (139.8987, 31.9182) centre (139.3987, 31.9182) ccw
  arc A267 (-39.9893, 27.8682) -> (-40.4893, 28.3682) centre (-40.4893, 27.8682) ccw
  line L207 (112.4107, 27.8682) -> (112.4107, 14.8682)
  arc A268 (159.5357, 33.4182) -> (160.0357, 33.9182) centre (159.5357, 33.9182) ccw
  line L208 (88.5982, -10.2318) -> (88.5982, -23.2318)
  line L209 (133.3987, 31.4182) -> (139.3987, 31.4182)
  line L210 (131.0174, 8.3182) -> (137.0174, 8.3182)
  line L211 (107.9357, 65.9682) -> (107.9357, 52.9682)
  line L212 (50.7857, 46.9182) -> (50.7857, 33.9182)
  arc A269 (107.9357, 52.9682) -> (108.4357, 52.4682) centre (108.4357, 52.9682) ccw
  line L213 (98.9107, 28.3682) -> (111.9107, 28.3682)
  arc A270 (146.0357, -42.2818) -> (146.5357, -42.7818) centre (146.5357, -42.2818) ccw
  arc A271 (160.0357, 27.8682) -> (159.5357, 28.3682) centre (159.5357, 27.8682) ccw
  arc A272 (121.4357, 52.4682) -> (121.9357, 52.9682) centre (121.4357, 52.9682) ccw
  line L214 (140.9857, 65.9682) -> (140.9857, 52.9682)
  line L215 (129.0794, 8.8182) -> (129.0794, -4.1818)
  line L216 (146.0357, 27.8682) -> (146.0357, 14.8682)
  line L217 (-113.0206, -28.7818) -> (-100.0206, -28.7818)
  arc A273 (117.4607, 33.9182) -> (117.9607, 33.4182) centre (117.9607, 33.9182) ccw
  line L218 (121.9357, 65.9682) -> (121.9357, 52.9682)
  line L219 (146.0357, 8.8182) -> (146.0357, -4.1818)
  line L220 (-105.8768, -4.6818) -> (-92.8768, -4.6818)
  arc A274 (146.0357, -23.2318) -> (146.5357, -23.7318) centre (146.5357, -23.2318) ccw
  arc A275 (160.0357, 8.8182) -> (159.5357, 9.3182) centre (159.5357, 8.8182) ccw
  line L221 (-35.2268, 8.8182) -> (-35.2268, -4.1818)
  line L222 (-96.8518, -10.2318) -> (-96.8518, -23.2318)
  arc A276 (140.9857, -10.2318) -> (140.4857, -9.7318) centre (140.4857, -10.2318) ccw
  line L223 (-82.8518, -10.2318) -> (-82.8518, -23.2318)
  arc A277 (126.9857, -42.2818) -> (127.4857, -42.7818) centre (127.4857, -42.2818) ccw
  arc A278 (137.5174, 7.8182) -> (137.0174, 8.3182) centre (137.0174, 7.8182) ccw
  arc A279 (137.0174, -6.6818) -> (137.5174, -6.1818) centre (137.0174, -6.1818) ccw
  arc A280 (69.0482, -23.7318) -> (69.5482, -23.2318) centre (69.0482, -23.2318) ccw
  line L224 (146.5357, 33.4182) -> (159.5357, 33.4182)
  line L225 (172.5639, -17.1628) -> (187.5639, -17.1628)
  line L226 (108.4357, 66.4682) -> (121.4357, 66.4682)
  arc A281 (45.2357, 33.4182) -> (45.7357, 33.9182) centre (45.2357, 33.9182) ccw
  line L227 (109.5227, 46.4182) -> (115.5227, 46.4182)
  line L228 (-15.8893, 65.9682) -> (-15.8893, 52.9682)
  line L229 (127.4857, -42.7818) -> (140.4857, -42.7818)
  arc A282 (102.3857, 52.4682) -> (102.8857, 52.9682) centre (102.3857, 52.9682) ccw
  line L230 (-39.2018, -9.7318) -> (-26.2018, -9.7318)
  arc A283 (135.7232, 14.3682) -> (136.2232, 14.8682) centre (135.7232, 14.8682) ccw
  arc A284 (-30.9643, 52.4682) -> (-30.4643, 52.9682) centre (-30.9643, 52.9682) ccw
  arc A285 (50.7857, 33.9182) -> (51.2857, 33.4182) centre (51.2857, 33.9182) ccw
  arc A286 (83.3357, -42.7818) -> (83.8357, -42.2818) centre (83.3357, -42.2818) ccw
  arc A287 (139.8987, 45.9182) -> (139.3987, 46.4182) centre (139.3987, 45.9182) ccw
  line L231 (-63.8018, -10.2318) -> (-63.8018, -23.2318)
  line L232 (-101.1143, 47.4182) -> (-88.1143, 47.4182)
  arc A288 (74.5982, -23.2318) -> (75.0982, -23.7318) centre (75.0982, -23.2318) ccw
  line L233 (136.2232, 27.8682) -> (136.2232, 14.8682)
  line L234 (146.5357, 14.3682) -> (159.5357, 14.3682)
  line L235 (137.5174, 7.8182) -> (137.5174, -6.1818)
  arc A289 (-30.1768, -4.1818) -> (-29.6768, -4.6818) centre (-29.6768, -4.1818) ccw
  arc A290 (100.7919, -23.2318) -> (101.2919, -23.7318) centre (101.2919, -23.2318) ccw
  arc A291 (88.0982, -23.7318) -> (88.5982, -23.2318) centre (88.0982, -23.2318) ccw
  arc A292 (-96.3518, -9.7318) -> (-96.8518, -10.2318) centre (-96.3518, -10.2318) ccw
  arc A293 (-129.7461, -25.7318) -> (-129.2461, -25.2318) centre (-129.7461, -25.2318) ccw
  arc A294 (136.2232, 27.8682) -> (135.7232, 28.3682) centre (135.7232, 27.8682) ccw
  arc A295 (-73.8268, -4.6818) -> (-73.3268, -4.1818) centre (-73.8268, -4.1818) ccw
  line L236 (126.9857, 65.9682) -> (126.9857, 52.9682)
  arc A296 (146.0357, 14.8682) -> (146.5357, 14.3682) centre (146.5357, 14.8682) ccw
  arc A297 (41.7607, 28.3682) -> (41.2607, 27.8682) centre (41.7607, 27.8682) ccw
  arc A298 (-34.9393, 14.8682) -> (-34.4393, 14.3682) centre (-34.4393, 14.8682) ccw
  line L237 (83.8357, -29.2818) -> (83.8357, -42.2818)
  arc A299 (-92.8768, -4.6818) -> (-92.3768, -4.1818) centre (-92.8768, -4.1818) ccw
  line L238 (45.7357, 46.9182) -> (45.7357, 33.9182)
  arc A300 (114.2919, -23.7318) -> (114.7919, -23.2318) centre (114.2919, -23.2318) ccw
  arc A301 (132.8987, 31.9182) -> (133.3987, 31.4182) centre (133.3987, 31.9182) ccw
  line L239 (133.3987, 46.4182) -> (139.3987, 46.4182)
  line L240 (121.9357, -29.2818) -> (121.9357, -42.2818)
  line L241 (146.5357, 9.3182) -> (159.5357, 9.3182)
  line L242 (-105.8768, 9.3182) -> (-92.8768, 9.3182)
  arc A302 (-112.3701, -25.2318) -> (-111.8701, -25.7318) centre (-111.8701, -25.2318) ccw
  arc A303 (129.0794, 8.8182) -> (128.5794, 9.3182) centre (128.5794, 8.8182) ccw
  arc A304 (121.9357, -29.2818) -> (121.4357, -28.7818) centre (121.4357, -29.2818) ccw
  arc A305 (159.5357, -4.6818) -> (160.0357, -4.1818) centre (159.5357, -4.1818) ccw
  arc A306 (88.8857, -42.2818) -> (89.3857, -42.7818) centre (89.3857, -42.2818) ccw
  arc A307 (128.5794, -4.6818) -> (129.0794, -4.1818) centre (128.5794, -4.1818) ccw
  line L243 (-77.8018, -10.2318) -> (-77.8018, -23.2318)
  arc A308 (127.4857, -28.7818) -> (126.9857, -29.2818) centre (127.4857, -29.2818) ccw
  line L244 (126.9857, -29.2818) -> (126.9857, -42.2818)
  arc A309 (-105.8701, -25.7318) -> (-105.3701, -25.2318) centre (-105.8701, -25.2318) ccw
  arc A310 (83.8357, -29.2818) -> (83.3357, -28.7818) centre (83.3357, -29.2818) ccw
  line L245 (-39.2018, -23.7318) -> (-26.2018, -23.7318)
  arc A311 (160.0357, -10.2318) -> (159.5357, -9.7318) centre (159.5357, -10.2318) ccw
  line L246 (187.5639, -32.1628) -> (172.5639, -32.1628)
  arc A312 (130.5174, -6.1818) -> (131.0174, -6.6818) centre (131.0174, -6.1818) ccw
  line L247 (-53.4893, 14.3682) -> (-40.4893, 14.3682)
  arc A313 (-26.2018, -23.7318) -> (-25.7018, -23.2318) centre (-26.2018, -23.2318) ccw
  line L248 (-57.7706, -30.2818) -> (-57.7706, -44.2818)
  line L249 (130.5174, 7.8182) -> (130.5174, -6.1818)
  arc A314 (131.4607, 46.9182) -> (130.9607, 47.4182) centre (130.9607, 46.9182) ccw
  arc A315 (-58.7518, -23.2318) -> (-58.2518, -23.7318) centre (-58.2518, -23.2318) ccw
  arc A316 (159.5357, -42.7818) -> (160.0357, -42.2818) centre (159.5357, -42.2818) ccw
  arc A317 (-87.3268, -4.1818) -> (-86.8268, -4.6818) centre (-86.8268, -4.1818) ccw
  line L250 (69.8357, -29.2818) -> (69.8357, -42.2818)
  arc A318 (107.1414, 8.3182) -> (106.6414, 7.8182) centre (107.1414, 7.8182) ccw
  line L251 (32.2357, 33.4182) -> (45.2357, 33.4182)
  arc A319 (-136.2461, -25.2318) -> (-135.7461, -25.7318) centre (-135.7461, -25.2318) ccw
  line L252 (55.2607, 27.8682) -> (55.2607, 14.8682)
  arc A320 (-4.2706, -29.2818) -> (-4.7706, -28.7818) centre (-4.7706, -29.2818) ccw
  line L253 (84.1232, 8.8182) -> (84.1232, -4.1818)
  line L254 (114.7919, -10.2318) -> (114.7919, -23.2318)
  line L255 (74.3107, 27.8682) -> (74.3107, 14.8682)
  arc A321 (-1.6018, -23.2318) -> (-1.1018, -23.7318) centre (-1.1018, -23.2318) ccw
  line L256 (17.1607, 27.8682) -> (17.1607, 14.8682)
  line L257 (-39.9893, 27.8682) -> (-39.9893, 14.8682)
  arc A322 (78.5732, -4.6818) -> (79.0732, -4.1818) centre (78.5732, -4.1818) ccw
  line L258 (-63.0143, 47.4182) -> (-50.0143, 47.4182)
  line L259 (117.9607, 33.4182) -> (130.9607, 33.4182)
  line L260 (-67.7768, 9.3182) -> (-54.7768, 9.3182)
  line L261 (122.7232, 28.3682) -> (135.7232, 28.3682)
  line L262 (60.3107, 27.8682) -> (60.3107, 14.8682)
  line L263 (22.2107, 27.8682) -> (22.2107, 14.8682)
  line L264 (-132.5706, 8.8182) -> (-132.5706, -4.1818)
  line L265 (-59.0393, 27.8682) -> (-59.0393, 14.8682)
  line L266 (-17.7706, -42.7818) -> (-4.7706, -42.7818)
  line L267 (108.4357, -28.7818) -> (121.4357, -28.7818)
  arc A323 (-17.7706, -28.7818) -> (-18.2706, -29.2818) centre (-17.7706, -29.2818) ccw
  line L268 (-15.8893, 27.8682) -> (-15.8893, 14.8682)
  line L269 (3.1607, 27.8682) -> (3.1607, 14.8682)
  line L270 (109.0227, 45.9182) -> (109.0227, 31.9182)
  line L271 (93.3607, 27.8682) -> (93.3607, 14.8682)
  line L272 (146.0357, -10.2318) -> (146.0357, -23.2318)
  line L273 (75.0982, -9.7318) -> (88.0982, -9.7318)
  arc A324 (79.3607, 14.8682) -> (79.8607, 14.3682) centre (79.8607, 14.8682) ccw
  line L274 (41.2607, 27.8682) -> (41.2607, 14.8682)
  line L275 (160.0357, 46.9182) -> (160.0357, 33.9182)
  line L276 (-53.9893, 27.8682) -> (-53.9893, 14.8682)
  line L277 (-87.3268, 8.8182) -> (-87.3268, -4.1818)
  line L278 (36.2107, 27.8682) -> (36.2107, 14.8682)
  line L279 (102.8857, 46.9182) -> (102.8857, 33.9182)
  line L280 (-1.8893, 27.8682) -> (-1.8893, 14.8682)
  line L281 (100.7919, -10.2318) -> (100.7919, -23.2318)
  line L282 (-68.2768, 8.8182) -> (-68.2768, -4.1818)
  line L283 (-34.9393, 27.8682) -> (-34.9393, 14.8682)
  line L284 (-6.6518, -10.2318) -> (-6.6518, -23.2318)
  line L285 (116.0227, 45.9182) -> (116.0227, 31.9182)
  line L286 (79.3607, 27.8682) -> (79.3607, 14.8682)
  line L287 (107.1414, 8.3182) -> (113.1414, 8.3182)
  line L288 (-20.9393, 27.8682) -> (-20.9393, 14.8682)
  line L289 (131.4607, 46.9182) -> (131.4607, 33.9182)
  line L290 (-34.4393, 28.3682) -> (-21.4393, 28.3682)
  line L291 (132.8987, 45.9182) -> (132.8987, 31.9182)
  line L292 (160.0357, -10.2318) -> (160.0357, -23.2318)
  arc A325 (84.1232, -4.1818) -> (84.6232, -4.6818) centre (84.6232, -4.1818) ccw
  line L293 (139.8987, 45.9182) -> (139.8987, 31.9182)
  arc A326 (98.4107, 14.8682) -> (98.9107, 14.3682) centre (98.9107, 14.8682) ccw
  line L294 (-73.3268, 8.8182) -> (-73.3268, -4.1818)
  line L295 (-20.6518, -10.2318) -> (-20.6518, -23.2318)
  arc A327 (117.9607, 47.4182) -> (117.4607, 46.9182) centre (117.9607, 46.9182) ccw
  line L296 (108.4357, 52.4682) -> (121.4357, 52.4682)
  line L297 (126.9857, -10.2318) -> (126.9857, -23.2318)
  line L298 (-24.9143, 33.4182) -> (-11.9143, 33.4182)
  line L299 (-106.3768, 8.8182) -> (-106.3768, -4.1818)
  arc A328 (111.9107, 14.3682) -> (112.4107, 14.8682) centre (111.9107, 14.8682) ccw
  arc A329 (60.0232, 8.8182) -> (59.5232, 9.3182) centre (59.5232, 8.8182) ccw
  line L300 (46.5232, 9.3182) -> (59.5232, 9.3182)
  line L301 (12.3982, -10.2318) -> (12.3982, -23.2318)
  line L302 (117.4607, 46.9182) -> (117.4607, 33.9182)
  line L303 (109.5227, 31.4182) -> (115.5227, 31.4182)
  line L304 (140.9857, -10.2318) -> (140.9857, -23.2318)
  arc A330 (102.8857, -29.2818) -> (102.3857, -28.7818) centre (102.3857, -29.2818) ccw
  line L305 (-1.6018, -10.2318) -> (-1.6018, -23.2318)
  line L306 (41.7607, 52.4682) -> (54.7607, 52.4682)
  line L307 (-29.6768, 9.3182) -> (-16.6768, 9.3182)
  arc A331 (109.5227, 46.4182) -> (109.0227, 45.9182) centre (109.5227, 45.9182) ccw
  line L308 (46.5232, -4.6818) -> (59.5232, -4.6818)
  arc A332 (69.5482, -10.2318) -> (69.0482, -9.7318) centre (69.0482, -10.2318) ccw
  arc A333 (79.0732, 8.8182) -> (78.5732, 9.3182) centre (78.5732, 8.8182) ccw
  arc A334 (102.8857, 65.9682) -> (102.3857, 66.4682) centre (102.3857, 65.9682) ccw
  line L309 (51.2857, 33.4182) -> (64.2857, 33.4182)
  line L310 (-92.3768, 8.8182) -> (-92.3768, -4.1818)
  line L311 (-29.6768, -4.6818) -> (-16.6768, -4.6818)
  line L312 (98.1232, 8.8182) -> (98.1232, -4.1818)
  arc A335 (65.5732, 9.3182) -> (65.0732, 8.8182) centre (65.5732, 8.8182) ccw
  line L313 (41.7607, 66.4682) -> (54.7607, 66.4682)
  arc A336 (115.0794, -4.1818) -> (115.5794, -4.6818) centre (115.5794, -4.1818) ccw
  arc A337 (97.6232, -4.6818) -> (98.1232, -4.1818) centre (97.6232, -4.1818) ccw
  line L314 (51.2857, -42.7818) -> (64.2857, -42.7818)
  arc A338 (115.5227, 31.4182) -> (116.0227, 31.9182) centre (115.5227, 31.9182) ccw
  line L315 (56.0482, -9.7318) -> (69.0482, -9.7318)
  arc A339 (121.9357, 65.9682) -> (121.4357, 66.4682) centre (121.4357, 65.9682) ccw
  line L316 (-24.9143, 47.4182) -> (-11.9143, 47.4182)
  line L317 (146.0357, 46.9182) -> (146.0357, 33.9182)
  line L318 (56.0482, -23.7318) -> (69.0482, -23.7318)
  arc A340 (73.8107, 14.3682) -> (74.3107, 14.8682) centre (73.8107, 14.8682) ccw
  arc A341 (108.4357, 66.4682) -> (107.9357, 65.9682) centre (108.4357, 65.9682) ccw
  line L319 (-118.5706, 8.8182) -> (-118.5706, -4.1818)
  line L320 (127.4857, -28.7818) -> (140.4857, -28.7818)
  line L321 (122.2232, 27.8682) -> (122.2232, 14.8682)
  line L322 (160.0357, -29.2818) -> (160.0357, -42.2818)
  line L323 (146.0357, -29.2818) -> (146.0357, -42.2818)
  line L324 (51.2857, -28.7818) -> (64.2857, -28.7818)
  line L325 (-34.4393, 14.3682) -> (-21.4393, 14.3682)
  arc A342 (98.9107, 28.3682) -> (98.4107, 27.8682) centre (98.9107, 27.8682) ccw
  line L326 (41.7607, 28.3682) -> (54.7607, 28.3682)
  arc A343 (113.6414, 7.8182) -> (113.1414, 8.3182) centre (113.1414, 7.8182) ccw
  line L327 (-63.0143, 66.4682) -> (-50.0143, 66.4682)
  arc A344 (65.0732, -4.1818) -> (65.5732, -4.6818) centre (65.5732, -4.1818) ccw
  line L328 (-1.1018, -23.7318) -> (11.8982, -23.7318)
  line L329 (89.3857, 52.4682) -> (102.3857, 52.4682)
  line L330 (89.3857, 47.4182) -> (102.3857, 47.4182)
  line L331 (79.8607, 14.3682) -> (92.8607, 14.3682)
  line L332 (84.6232, 9.3182) -> (97.6232, 9.3182)
  arc A345 (-20.6518, -23.2318) -> (-20.1518, -23.7318) centre (-20.1518, -23.2318) ccw
  line L333 (-72.5393, 28.3682) -> (-59.5393, 28.3682)
  arc A346 (59.5232, -4.6818) -> (60.0232, -4.1818) centre (59.5232, -4.1818) ccw
  line L334 (-20.1518, -23.7318) -> (-7.1518, -23.7318)
  line L335 (79.0732, 8.8182) -> (79.0732, -4.1818)
  line L336 (-72.5393, 14.3682) -> (-59.5393, 14.3682)
  arc A347 (-18.2706, -42.2818) -> (-17.7706, -42.7818) centre (-17.7706, -42.2818) ccw
  line L337 (117.9607, 47.4182) -> (130.9607, 47.4182)
  arc A348 (60.3107, 14.8682) -> (60.8107, 14.3682) centre (60.8107, 14.8682) ccw
  line L338 (65.5732, 9.3182) -> (78.5732, 9.3182)
  line L339 (-18.2706, -29.2818) -> (-18.2706, -42.2818)
  line L340 (115.5794, -4.6818) -> (128.5794, -4.6818)
  line L341 (212.5639, 86.0492) -> (212.5639, -64.1628)
  line L342 (115.5794, 9.3182) -> (128.5794, 9.3182)
  line L343 (-64.2706, -29.7818) -> (-58.2706, -29.7818)
  line L344 (122.7232, 14.3682) -> (135.7232, 14.3682)
  line L345 (31.4482, -10.2318) -> (31.4482, -23.2318)
  line L346 (-10.6268, -4.6818) -> (2.3732, -4.6818)
  line L347 (-20.1518, -9.7318) -> (-7.1518, -9.7318)
  line L348 (17.4482, -10.2318) -> (17.4482, -23.2318)
  arc A349 (12.3982, -10.2318) -> (11.8982, -9.7318) centre (11.8982, -10.2318) ccw
  arc A350 (2.3732, -4.6818) -> (2.8732, -4.1818) centre (2.3732, -4.1818) ccw
  line L349 (2.8732, 8.8182) -> (2.8732, -4.1818)
  line L350 (50.4982, -10.2318) -> (50.4982, -23.2318)
  line L351 (-10.6268, 9.3182) -> (2.3732, 9.3182)
  arc A351 (56.0482, -9.7318) -> (55.5482, -10.2318) centre (56.0482, -10.2318) ccw
  arc A352 (46.0232, -4.1818) -> (46.5232, -4.6818) centre (46.5232, -4.1818) ccw
  arc A353 (21.4232, -4.6818) -> (21.9232, -4.1818) centre (21.4232, -4.1818) ccw
  line L352 (36.9982, -9.7318) -> (49.9982, -9.7318)
  line L353 (89.3857, -42.7818) -> (102.3857, -42.7818)
  arc A354 (88.5982, -10.2318) -> (88.0982, -9.7318) centre (88.0982, -10.2318) ccw
  line L354 (65.5732, -4.6818) -> (78.5732, -4.6818)
  arc A355 (-4.7706, -42.7818) -> (-4.2706, -42.2818) centre (-4.7706, -42.2818) ccw
  line L355 (-63.0143, 33.4182) -> (-50.0143, 33.4182)
  line L356 (65.0732, 8.8182) -> (65.0732, -4.1818)
  line L357 (60.0232, 8.8182) -> (60.0232, -4.1818)
  arc A356 (-7.1518, -23.7318) -> (-6.6518, -23.2318) centre (-7.1518, -23.2318) ccw
  arc A357 (11.8982, -23.7318) -> (12.3982, -23.2318) centre (11.8982, -23.2318) ccw